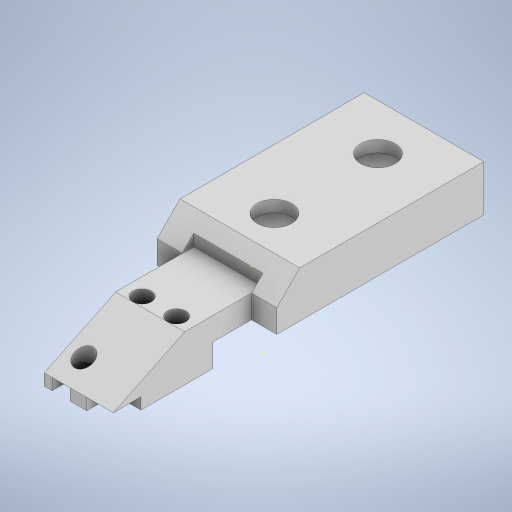
# Autodesk Inventor part: electrodeholder_screwon_4
Saved by Autodesk Inventor 2023 (Build 270158000, 158)
## iProperties
Created: 2022-09-20
Part Number: electrodeholder_screwon_4
Material: Generic
Document SubType Name: Modeling
Designer: Connor
Density: 1 g/cm^3
Appearance: Default
Author: Connor
Autodesk Inventor part; units mm, degrees
ref_plane "YZ Plane" through (0, 0, 0) normal (1, 0, 0) x (0, 1, 0)
ref_plane "XZ Plane" through (0, 0, 0) normal (0, 1, 0) x (-1, 0, 0)
ref_plane "XY Plane" through (0, 0, 0) normal (0, 0, 1) x (1, 0, 0)
sketch "Sketch1" plane through (0, 0, 0) normal (0, 1, 0) x (-1, 0, 0)
  line L0 (0, 0) -> (12.7, 0)
  line L1 (12.7, 0) -> (12.7, -25.4)
  line L2 (12.7, -25.4) -> (0, -25.4)
  line L3 (0, -25.4) -> (0, 0)
  dimension "d0" = 12.7
  dimension "d1" = 25.4
  constraints: 8 end point, 2 parallel, 1 horizontal, 1 perpendicular
  measures "d0" distance of L1.end L2.end
  measures "d1" distance of L0.end L1.end
sketch "Sketch1 outline for Extrusion1" plane through (0, 0, 0) normal (0, 1, 0) x (-1, 0, 0)
  line L0 (0, 0) -> (0, -25.4)
  line L1 (12.7, 0) -> (0, 0)
  line L2 (12.7, -25.4) -> (12.7, 0)
  line L3 (0, -25.4) -> (12.7, -25.4)
extrude "Extrusion1" add sketch "Sketch1 outline for Extrusion1" along normal blind 7.62
sketch "Sketch2" plane through (0, 0, 0) normal (1, 0, 0) x (0, 0, -1)
  line L0 (25.4, 7.62) -> (0, 7.62) projected
  line L1 (25.4, 0) -> (0, 0) projected
  line L2 (0, 7.62) -> (7.62, 7.62)
  line L3 (7.62, 7.62) -> (7.62, 0)
  line L4 (7.62, 0) -> (0, 0)
  line L5 (0, 0) -> (0, 7.62)
  line L6 (0, 0) -> (7.62, 7.62)
  dimension "d4" = 7.62
  constraints: 10 end point, 2 parallel, 1 horizontal, 1 perpendicular, 1 point on line
  measures "d4" distance of L3.end L4.end
sketch "Sketch2 outline for Extrusion2" plane through (0, 0, 0) normal (1, 0, 0) x (0, 0, -1)
  line L0 (0, 7.62) -> (0, 0)
  line L1 (7.62, 7.62) -> (0, 7.62)
  line L2 (0, 0) -> (7.62, 7.62)
extrude "Extrusion2" cut sketch "Sketch2 outline for Extrusion2" against normal blind 25.4
sketch "Sketch3" plane through (0, 0, 0) normal (0, -1, 0) x (1, 0, 0)
  line L0 (-12.7, -25.4) -> (-12.7, 0) projected
  line L1 (0, 0) -> (-12.7, 0)
  line L2 (-12.7, 0) -> (-12.7, -8.89)
  line L3 (-12.7, -8.89) -> (0, -8.89)
  line L4 (0, -8.89) -> (0, 0)
  circle A0 centre (-6.35, -8.89) radius 4.445
  dimension "d7" = 8.89
  dimension "d8" = 8.89
  constraints: 8 end point, 2 parallel, 1 centre point, 1 horizontal, 1 midpoint, 1 perpendicular, 1 point on line
  measures "d7" distance of L2.end L1.end
  measures "d8" diameter of A0
sketch "Sketch3 outline for Extrusion3" plane through (0, 0, 0) normal (0, -1, 0) x (1, 0, 0)
  circle A0 centre (-6.35, -8.89) radius 4.445
extrude "Extrusion3" cut sketch "Sketch3 outline for Extrusion3" against normal blind 3.81
sketch "Sketch4" plane through (0, 0, 0) normal (0, -1, 0) x (1, 0, 0)
  circle A0 centre (-6.35, -8.89) radius 4.445 projected
  line L0 (-6.35, -8.89) -> (-6.35, -20.32)
  circle A1 centre (-6.35, -20.32) radius 4.445
  point P0 (0, 0)
  dimension "d11" = 11.43
  dimension "d12" = 8.89
  constraints: 2 end point, 1 centre point, 1 coincident, 1 vertical
  measures "d11" distance of L0.start L0.end
  measures "d12" diameter of A1
sketch "Sketch4 outline for Extrusion4" plane through (0, 0, 0) normal (0, -1, 0) x (1, 0, 0)
  circle A0 centre (-6.35, -20.32) radius 4.445
extrude "Extrusion4" cut sketch "Sketch4 outline for Extrusion4" against normal blind 2.54
sketch "Sketch6" plane through (0, 0, -25.4) normal (1, 0, 0) x (0, 0, -1)
  line L0 (-25.4, 0) -> (-22.86, 0)
  line L1 (-22.86, 0) -> (-22.86, 2.54)
  line L2 (-22.86, 2.54) -> (-25.4, 2.54)
  line L3 (-25.4, 2.54) -> (-25.4, 0)
  dimension "d18" = 2.54
  dimension "d19" = 2.54
  constraints: 8 end point, 2 parallel, 1 horizontal, 1 perpendicular
  measures "d18" distance of L2.end L1.end
  measures "d19" distance of L1.end L0.end
sketch "Sketch6 outline for Extrusion6" plane through (0, 0, -25.4) normal (1, 0, 0) x (0, 0, -1)
  line L0 (-25.4, 0) -> (-22.86, 0)
  line L1 (-25.4, 2.54) -> (-25.4, 0)
  line L2 (-22.86, 2.54) -> (-25.4, 2.54)
  line L3 (-22.86, 0) -> (-22.86, 2.54)
extrude "Extrusion6" cut sketch "Sketch6 outline for Extrusion6" against normal blind 25.4
sketch "Sketch7" plane through (0, 0, -2.54) normal (0, 0, 1) x (1, 0, 0)
  line L0 (-12.7, 0) -> (-12.7, 2.54) projected
  line L1 (0, 0) -> (-12.7, 0) projected
  line L2 (0, 2.54) -> (0, 0) projected
  line L3 (-12.7, 2.54) -> (0, 2.54) projected
sketch "Sketch7 outline for Extrusion7" plane through (0, 0, -2.54) normal (0, 0, 1) x (1, 0, 0)
  line L0 (-12.7, 0) -> (0, 0)
  line L1 (-12.7, 2.54) -> (-12.7, 0)
  line L2 (0, 2.54) -> (-12.7, 2.54)
  line L3 (0, 0) -> (0, 2.54)
extrude "Extrusion7" add sketch "Sketch7 outline for Extrusion7" along normal blind 12.7
sketch "Sketch13" plane through (0, 0, 0) normal (0, -1, 0) x (1, 0, 0)
  line L0 (-12.7, -2.54) -> (-12.7, -7.62) projected
  line L1 (0, -2.54) -> (0, 10.16) projected
  line L2 (-12.7, -2.54) -> (0, -2.54)
  line L3 (0, -2.54) -> (0, 10.16)
  line L4 (0, 10.16) -> (-12.7, 10.16)
  line L5 (-12.7, 10.16) -> (-12.7, -2.54)
  line L6 (0, -7.62) -> (0, -2.54) projected
  line L7 (-12.7, 10.16) -> (0, 10.16) projected
  line L8 (0, -2.54) -> (-2.54, -2.54)
  line L9 (-2.54, -2.54) -> (-2.54, 10.16)
  line L10 (-2.54, 10.16) -> (0, 10.16)
  line L11 (0, 10.16) -> (0, -2.54)
  line L12 (-12.7, -2.54) -> (-10.16, -2.54)
  line L13 (-10.16, -2.54) -> (-10.16, 10.16)
  line L14 (-10.16, 10.16) -> (-12.7, 10.16)
  line L15 (-12.7, 10.16) -> (-12.7, -2.54)
  point P0 (0, 0)
  dimension "d43" = 2.54
  dimension "d44" = 2.54
  constraints: 24 end point, 6 parallel, 3 horizontal, 3 perpendicular, 2 point on line
  measures "d43" distance of L9.end L10.end
  measures "d44" distance of L14.end L13.end
sketch "Sketch13 outline for Extrusion13" plane through (0, 0, 0) normal (0, -1, 0) x (1, 0, 0)
  line L0 (-10.16, -2.54) -> (-10.16, 10.16)
  line L1 (-12.7, -2.54) -> (-10.16, -2.54)
  line L2 (-12.7, 10.16) -> (-12.7, -2.54)
  line L3 (-10.16, 10.16) -> (-12.7, 10.16)
  line L4 (-2.54, 10.16) -> (-2.54, -2.54)
  line L5 (0, 10.16) -> (-2.54, 10.16)
  line L6 (0, -2.54) -> (0, 10.16)
  line L7 (-2.54, -2.54) -> (0, -2.54)
extrude "Extrusion13" cut sketch "Sketch13 outline for Extrusion13" against normal blind 2.54
sketch "Sketch18" plane through (0, 0, 0) normal (0, -1, 0) x (1, 0, 0)
  line L0 (-2.54, 10.16) -> (-10.16, 10.16) projected
  line L1 (-10.16, -2.54) -> (-10.16, 10.16) projected
  line L2 (-2.54, 10.16) -> (-10.16, 10.16)
  line L3 (-10.16, 10.16) -> (-10.16, 2.54)
  line L4 (-10.16, 2.54) -> (-2.54, 2.54)
  line L5 (-2.54, 2.54) -> (-2.54, 10.16)
  line L6 (-10.16, -2.54) -> (-2.54, -2.54) projected
  line L7 (-6.35, -2.54) -> (-6.35, 10.16)
  line L8 (-6.35, -2.54) -> (-2.54, -2.54)
  line L9 (-2.54, -2.54) -> (-4.445, -2.54)
  line L10 (-4.445, 10.16) -> (-4.445, -2.54)
  line L11 (-10.16, -2.54) -> (-6.35, -2.54)
  line L12 (-8.255, -2.54) -> (-8.255, 10.16)
  circle A0 centre (-4.445, 3.81) radius 1.016
  circle A1 centre (-8.255, 3.81) radius 1.016
  point P0 (0, 0)
  dimension "d63" = 7.62
  dimension "d64" = 2.032
  dimension "d65" = 2.032
  constraints: 20 end point, 6 midpoint, 4 perpendicular, 3 point on line, 2 centre point, 2 horizontal, 2 parallel
  measures "d63" distance of L3.end L2.end
  measures "d64" diameter of A0
  measures "d65" diameter of A1
sketch "Sketch18 outline for Extrusion18" plane through (0, 0, 0) normal (0, -1, 0) x (1, 0, 0)
  circle A0 centre (-8.255, 3.81) radius 1.016
  circle A1 centre (-4.445, 3.81) radius 1.016
extrude "Extrusion18" cut sketch "Sketch18 outline for Extrusion18" against normal blind 25.4
sketch "Sketch19" plane through (0, 0, 0) normal (0, -1, 0) x (1, 0, 0)
  circle A0 centre (-4.445, 3.81) radius 1.016
  line L0 (-2.54, 10.16) -> (-10.16, 10.16)
  line L1 (-5.461, 3.81) -> (-7.285663, 3.81)
  line L2 (-7.285663, 3.81) -> (-7.285663, 10.16)
  line L3 (-7.285663, 10.16) -> (-5.461, 10.16)
  line L4 (-5.461, 10.16) -> (-5.461, 3.81)
  point P0 (0, 0)
  constraints: 8 end point, 2 parallel, 1 horizontal, 1 horizontal alignment, 1 perpendicular, 1 point on line, 1 other
sketch "Sketch19 outline for Extrusion19" plane through (0, 0, 0) normal (0, -1, 0) x (1, 0, 0)
  line L0 (-5.461, 3.81) -> (-5.461, 10.16)
  line L1 (-7.285663, 3.81) -> (-5.461, 3.81)
  line L2 (-7.285663, 10.16) -> (-7.285663, 3.81)
  line L3 (-5.461, 10.16) -> (-7.285663, 10.16)
extrude "Extrusion19" add sketch "Sketch19 outline for Extrusion19" along normal blind 2.54
sketch "Sketch20" plane through (0, 0, 0) normal (0, -1, 0) x (1, 0, 0)
  line L0 (-5.461, 3.81) -> (-7.239, 3.81) projected
  line L1 (-5.461, 3.81) -> (-7.239, 3.81)
  line L2 (-7.239, 3.81) -> (-7.239, 2.54)
  line L3 (-7.239, 2.54) -> (-5.461, 2.54)
  line L4 (-5.461, 2.54) -> (-5.461, 3.81)
  point P0 (0, 0)
  dimension "d70" = 1.27
  constraints: 8 end point, 2 parallel, 1 horizontal, 1 perpendicular
  measures "d70" distance of L2.end L1.end
sketch "Sketch20 outline for Extrusion20" plane through (0, 0, 0) normal (0, -1, 0) x (1, 0, 0)
  line L0 (-5.461, 2.54) -> (-5.461, 3.81)
  line L1 (-7.239, 2.54) -> (-5.461, 2.54)
  line L2 (-7.239, 3.81) -> (-7.239, 2.54)
  line L3 (-5.461, 3.81) -> (-7.239, 3.81)
extrude "Extrusion20" add sketch "Sketch20 outline for Extrusion20" along normal blind 2.54
sketch "Sketch21" plane through (-10.16, 2.54, 10.16) normal (0, 1, 0) x (1, 0, 0)
  circle A0 centre (1.905, 6.35) radius 1.016 projected
  circle A1 centre (5.715, 6.35) radius 1.016 projected
  line L0 (0, 12.7) -> (0, 0) projected
  line L1 (7.62, 0) -> (0, 0) projected
  line L2 (7.62, 0) -> (7.62, 12.7) projected
  line L3 (0, 12.7) -> (7.62, 12.7) projected
  point P0 (10.16, 10.16)
sketch "Sketch21 outline for Extrusion21" plane through (-10.16, 2.54, 10.16) normal (0, 1, 0) x (1, 0, 0)
  line L0 (7.62, 0) -> (7.62, 12.7)
  line L1 (0, 0) -> (7.62, 0)
  line L2 (7.62, 12.7) -> (0, 12.7)
  line L3 (0, 12.7) -> (0, 0)
  circle A0 centre (1.905, 6.35) radius 1.016
  circle A1 centre (5.715, 6.35) radius 1.016
extrude "Extrusion21" add sketch "Sketch21 outline for Extrusion21" along normal blind 1.27
sketch "Sketch22" plane through (-2.54, 2.54, -2.54) normal (0, 0, -1) x (-1, 0, 0)
  line L0 (7.62, 0) -> (0, 0) projected
  line L1 (7.62, 0) -> (7.62, 1.27) projected
  line L2 (0, 1.27) -> (7.62, 1.27) projected
  line L3 (0, 0) -> (0, 1.27) projected
  point P0 (-2.54, -2.54)
sketch "Sketch22 outline for Extrusion22" plane through (-2.54, 2.54, -2.54) normal (0, 0, -1) x (-1, 0, 0)
  line L0 (7.62, 0) -> (7.62, 1.27)
  line L1 (0, 0) -> (7.62, 0)
  line L2 (0, 1.27) -> (0, 0)
  line L3 (7.62, 1.27) -> (0, 1.27)
extrude "Extrusion22" add sketch "Sketch22 outline for Extrusion22" along normal blind 5.08
sketch "Sketch23" plane through (-6.35, 2.54, -8.89) normal (0, -1, 0) x (1, 0, 0)
  circle A0 centre (0, 0) radius 4.445
  point P0 (6.35, 8.89)
  constraints: 1 centre point
sketch "Sketch23 outline for Extrusion23" plane through (-6.35, 2.54, -8.89) normal (0, -1, 0) x (1, 0, 0)
  circle A0 centre (0, 0) radius 4.445
extrude "Extrusion23" cut sketch "Sketch23 outline for Extrusion23" against normal blind 1.27
sketch "Sketch24" plane through (-10.16, 3.81, 10.16) normal (0, 1, 0) x (1, 0, 0)
  line L0 (0, 0) -> (0, 13.97) projected
  line L1 (0, 0) -> (7.62, 0) projected
  line L2 (7.62, 0) -> (7.62, 13.97) projected
  line L3 (0, 13.97) -> (7.62, 13.97) projected
  circle A0 centre (5.715, 6.35) radius 1.016 projected
  circle A1 centre (1.905, 6.35) radius 1.016 projected
  point P0 (10.16, 10.16)
sketch "Sketch24 outline for Extrusion24" plane through (-10.16, 3.81, 10.16) normal (0, 1, 0) x (1, 0, 0)
  line L0 (7.62, 0) -> (7.62, 13.97)
  line L1 (0, 0) -> (7.62, 0)
  line L2 (7.62, 13.97) -> (0, 13.97)
  line L3 (0, 13.97) -> (0, 0)
  circle A0 centre (1.905, 6.35) radius 1.016
  circle A1 centre (5.715, 6.35) radius 1.016
extrude "Extrusion24" cut sketch "Sketch24 outline for Extrusion24" against normal blind 2.54
sketch "Sketch26" plane through (0, 0, 10.16) normal (0, 0, 1) x (1, 0, 0)
  line L0 (-2.54, 1.27) -> (-10.16, 1.27)
  line L1 (-10.16, 0) -> (-10.16, 1.27)
  line L2 (-10.16, 0) -> (-7.285663, 0)
  line L3 (-7.285663, 0) -> (-7.285663, -2.54)
  line L4 (-5.461, -2.54) -> (-7.285663, -2.54)
  line L5 (-5.461, 0) -> (-5.461, -2.54)
  line L6 (-5.461, 0) -> (-2.54, 0)
  line L7 (-2.54, 0) -> (-2.54, 1.27)
  point P0 (0, 0)
sketch "Sketch26 outline for Extrusion26" plane through (0, 0, 10.16) normal (0, 0, 1) x (1, 0, 0)
  line L0 (-5.461, 0) -> (-2.54, 0)
  line L1 (-5.461, -2.54) -> (-5.461, 0)
  line L2 (-7.285663, -2.54) -> (-5.461, -2.54)
  line L3 (-7.285663, 0) -> (-7.285663, -2.54)
  line L4 (-10.16, 0) -> (-7.285663, 0)
  line L5 (-10.16, 1.27) -> (-10.16, 0)
  line L6 (-2.54, 1.27) -> (-10.16, 1.27)
  line L7 (-2.54, 0) -> (-2.54, 1.27)
extrude "Extrusion26" add sketch "Sketch26 outline for Extrusion26" along normal blind 2.54
sketch "Sketch27" plane through (0, 0, -25.4) normal (1, 0, 0) x (0, 0, -1)
  line L0 (-22.86, 2.54) -> (-22.86, 0) projected
  line L1 (-22.86, 0) -> (0, 0) projected
  line L2 (0, 0) -> (0, 7.62) projected
  line L3 (-17.78, 7.62) -> (0, 7.62) projected
  line L4 (-17.78, 7.62) -> (-22.86, 2.54) projected
  point P0 (-25.4, 0)
sketch "Sketch27 outline for Extrusion27" plane through (0, 0, -25.4) normal (1, 0, 0) x (0, 0, -1)
  line L0 (-17.78, 7.62) -> (-22.86, 2.54)
  line L1 (0, 7.62) -> (-17.78, 7.62)
  line L2 (0, 0) -> (0, 7.62)
  line L3 (-22.86, 0) -> (0, 0)
  line L4 (-22.86, 2.54) -> (-22.86, 0)
extrude "Extrusion27" add sketch "Sketch27 outline for Extrusion27" along normal blind 1.27
sketch "Sketch28" plane through (-12.7, 0, -25.4) normal (-1, 0, 0) x (0, 0, 1)
  line L0 (0, 7.62) -> (17.78, 7.62) projected
  line L1 (0, 0) -> (0, 7.62) projected
  line L2 (0, 0) -> (22.86, 0) projected
  line L3 (22.86, 0) -> (22.86, 2.54) projected
  line L4 (22.86, 2.54) -> (17.78, 7.62) projected
  point P0 (25.4, 0)
sketch "Sketch28 outline for Extrusion28" plane through (-12.7, 0, -25.4) normal (-1, 0, 0) x (0, 0, 1)
  line L0 (0, 0) -> (22.86, 0)
  line L1 (0, 7.62) -> (0, 0)
  line L2 (17.78, 7.62) -> (0, 7.62)
  line L3 (22.86, 2.54) -> (17.78, 7.62)
  line L4 (22.86, 0) -> (22.86, 2.54)
extrude "Extrusion28" add sketch "Sketch28 outline for Extrusion28" along normal blind 1.27
sketch "Sketch29" plane through (0, -2.54, 0) normal (0, -1, 0) x (1, 0, 0)
  line L0 (-7.285663, 3.81) -> (-7.285663, 12.7)
  line L1 (-7.285663, 3.81) -> (-7.239, 3.81)
  line L2 (-7.239, 3.81) -> (-7.239, 2.54)
  line L3 (-7.239, 2.54) -> (-5.461, 2.54)
  line L4 (-5.461, 2.54) -> (-5.461, 12.7)
  line L5 (-7.285663, 12.7) -> (-5.461, 12.7)
  point P0 (0, 0)
sketch "Sketch29 outline for Extrusion29" plane through (0, -2.54, 0) normal (0, -1, 0) x (1, 0, 0)
  line L0 (-7.239, 3.81) -> (-7.239, 2.54)
  line L1 (-7.285663, 3.81) -> (-7.239, 3.81)
  line L2 (-7.285663, 12.7) -> (-7.285663, 3.81)
  line L3 (-5.461, 12.7) -> (-7.285663, 12.7)
  line L4 (-5.461, 2.54) -> (-5.461, 12.7)
  line L5 (-7.239, 2.54) -> (-5.461, 2.54)
extrude "Extrusion29" cut sketch "Sketch29 outline for Extrusion29" against normal blind 1.27
sketch "Sketch31" plane through (0, 7.62, 0) normal (0, 1, 0) x (1, 0, 0)
  point P0 (0, 0)
sketch "Sketch32" plane through (0, 7.62, 0) normal (0, 1, 0) x (1, 0, 0)
  point P0 (0, 0)
sketch "Sketch33" plane through (0, 7.62, 0) normal (0, 1, 0) x (1, 0, 0)
  line L0 (-13.97, 7.62) -> (1.27, 7.62) projected
  line L1 (1.27, 25.4) -> (1.27, 7.62) projected
  line L2 (-13.97, 25.4) -> (1.27, 25.4) projected
  line L3 (-13.97, 7.62) -> (-13.97, 25.4) projected
  point P0 (0, 0)
sketch "Sketch33 outline for Extrusion30" plane through (0, 7.62, 0) normal (0, 1, 0) x (1, 0, 0)
  line L0 (-13.97, 25.4) -> (-13.97, 7.62)
  line L1 (1.27, 25.4) -> (-13.97, 25.4)
  line L2 (1.27, 7.62) -> (1.27, 25.4)
  line L3 (-13.97, 7.62) -> (1.27, 7.62)
extrude "Extrusion30" add sketch "Sketch33 outline for Extrusion30" along normal blind 5.08
sketch "Sketch35" plane through (1.27, 0, -25.4) normal (1, 0, 0) x (0, 0, -1)
  point P0 (-25.4, 0)
sketch "Sketch36" plane through (1.27, 0, -25.4) normal (1, 0, 0) x (0, 0, -1)
  line L0 (-22.86, 2.54) -> (-22.86, 0) projected
  line L1 (-22.86, 0) -> (0, 0) projected
  line L2 (0, 0) -> (0, 12.7) projected
  line L3 (-17.78, 12.7) -> (0, 12.7) projected
  line L4 (-17.78, 7.62) -> (-17.78, 12.7) projected
  line L5 (-17.78, 7.62) -> (-22.86, 2.54) projected
  point P0 (-25.4, 0)
sketch "Sketch36 outline for Extrusion33" plane through (1.27, 0, -25.4) normal (1, 0, 0) x (0, 0, -1)
  line L0 (-17.78, 7.62) -> (-22.86, 2.54)
  line L1 (-17.78, 12.7) -> (-17.78, 7.62)
  line L2 (0, 12.7) -> (-17.78, 12.7)
  line L3 (0, 0) -> (0, 12.7)
  line L4 (-22.86, 0) -> (0, 0)
  line L5 (-22.86, 2.54) -> (-22.86, 0)
extrude "Extrusion33" cut sketch "Sketch36 outline for Extrusion33" against normal blind 0.254
sketch "Sketch37" plane through (-13.97, 0, -25.4) normal (-1, 0, 0) x (0, 0, 1)
  line L0 (22.86, 0) -> (22.86, 2.54) projected
  line L1 (22.86, 2.54) -> (17.78, 7.62) projected
  line L2 (17.78, 7.62) -> (17.78, 12.7) projected
  line L3 (0, 12.7) -> (17.78, 12.7) projected
  line L4 (0, 0) -> (0, 12.7) projected
  line L5 (0, 0) -> (22.86, 0) projected
  point P0 (25.4, 0)
sketch "Sketch37 outline for Extrusion34" plane through (-13.97, 0, -25.4) normal (-1, 0, 0) x (0, 0, 1)
  line L0 (0, 0) -> (22.86, 0)
  line L1 (0, 12.7) -> (0, 0)
  line L2 (17.78, 12.7) -> (0, 12.7)
  line L3 (17.78, 7.62) -> (17.78, 12.7)
  line L4 (22.86, 2.54) -> (17.78, 7.62)
  line L5 (22.86, 0) -> (22.86, 2.54)
extrude "Extrusion34" cut sketch "Sketch37 outline for Extrusion34" against normal blind 0.254
sketch "Sketch38" plane through (0, 0, 0) normal (0, -1, 0) x (1, 0, 0)
  line L0 (-10.16, -2.54) -> (-10.16, 12.7)
  line L1 (-2.54, -2.54) -> (-2.54, 12.7)
  line L2 (-10.16, 12.7) -> (-2.54, 12.7)
  line L3 (-2.54, 12.7) -> (-2.54, 1.734585)
  line L4 (-2.54, 1.734585) -> (-10.16, 1.734585)
  line L5 (-10.16, 1.734585) -> (-10.16, 12.7)
  circle A0 centre (-6.35, -8.89) radius 4.445
  circle A1 centre (-6.35, -20.32) radius 4.445
  line L6 (-13.716, -2.54) -> (-13.716, -25.4)
  line L7 (1.016, -25.4) -> (-13.716, -25.4)
  line L8 (1.016, -25.4) -> (1.016, -2.54)
  line L9 (1.016, -2.54) -> (-2.54, -2.54)
  line L10 (-2.54, -2.54) -> (-2.54, 12.7)
  line L11 (-5.461, 12.7) -> (-2.54, 12.7)
  line L12 (-5.461, 12.7) -> (-5.461, 3.81)
  circle A2 centre (-4.445, 3.81) radius 1.016
  line L13 (-5.461, 3.81) -> (-5.461, 2.54)
  line L14 (-5.461, 2.54) -> (-7.239, 2.54)
  line L15 (-7.239, 2.54) -> (-7.239, 3.81)
  arc A3 (-7.285663, 4.114372) -> (-7.239, 3.81) centre (-8.255, 3.81) ccw
  line L16 (-7.285663, 4.114372) -> (-7.285663, 12.7)
  line L17 (-10.16, 12.7) -> (-7.285663, 12.7)
  line L18 (-10.16, 12.7) -> (-10.16, -2.54)
  line L19 (-10.16, -2.54) -> (-13.716, -2.54)
  point P0 (0, 0)
  constraints: 8 end point, 2 parallel, 1 horizontal, 1 horizontal alignment, 1 perpendicular, 1 point on line
sketch "Sketch38 outline for Extrusion35" plane through (0, 0, 0) normal (0, -1, 0) x (1, 0, 0)
  line L0 (-5.461, 2.54) -> (-7.239, 2.54)
  line L1 (-5.461, 3.81) -> (-5.461, 2.54)
  line L2 (-5.461, 12.7) -> (-5.461, 3.81)
  line L3 (-2.54, 12.7) -> (-5.461, 12.7)
  line L4 (-2.54, 1.734585) -> (-2.54, 12.7)
  line L5 (-10.16, 1.734585) -> (-2.54, 1.734585)
  line L6 (-10.16, 12.7) -> (-10.16, 1.734585)
  line L7 (-7.285663, 12.7) -> (-10.16, 12.7)
  line L8 (-7.285663, 4.114372) -> (-7.285663, 12.7)
  arc A0 (-7.239, 3.81) -> (-7.285663, 4.114372) centre (-8.255, 3.81) cw
  line L9 (-7.239, 2.54) -> (-7.239, 3.81)
  arc A1 (-5.461, 3.81) -> (-3.429, 3.81) centre (-4.445, 3.81) ccw
  arc A2 (-3.429, 3.81) -> (-5.461, 3.81) centre (-4.445, 3.81) ccw
extrude "Extrusion35" add sketch "Sketch38 outline for Extrusion35" along normal blind 1.27
sketch "Sketch39" plane through (0, -1.27, 0) normal (0, -1, 0) x (1, 0, 0)
  line L0 (-2.54, 12.7) -> (-10.16, 12.7)
  line L1 (-5.462315, 3.81) -> (-7.300103, 3.81)
  line L2 (-7.300103, 3.81) -> (-7.300103, 12.7)
  line L3 (-7.300103, 12.7) -> (-5.462315, 12.7)
  line L4 (-5.462315, 12.7) -> (-5.462315, 3.81)
  point P0 (0, 0)
  constraints: 8 end point, 2 parallel, 1 horizontal, 1 perpendicular, 1 point on line
sketch "Sketch39 outline for Extrusion36" plane through (0, -1.27, 0) normal (0, -1, 0) x (1, 0, 0)
  line L0 (-7.300103, 3.81) -> (-5.462315, 3.81)
  line L1 (-7.300103, 12.7) -> (-7.300103, 3.81)
  line L2 (-5.462315, 12.7) -> (-7.300103, 12.7)
  line L3 (-5.462315, 3.81) -> (-5.462315, 12.7)
extrude "Extrusion36" add sketch "Sketch39 outline for Extrusion36" along normal blind 1.27
sketch "Sketch40" plane through (0, -1.27, 0) normal (0, -1, 0) x (1, 0, 0)
  circle A0 centre (-4.445, 3.81) radius 1.016
  line L0 (-5.461, 3.81) -> (-7.300103, 3.81)
  line L1 (-7.300103, 3.81) -> (-7.300103, 2.501434)
  line L2 (-7.300103, 2.501434) -> (-5.461, 2.501434)
  line L3 (-5.461, 2.501434) -> (-5.461, 3.81)
  point P0 (0, 0)
  constraints: 8 end point, 2 parallel, 1 horizontal, 1 horizontal alignment, 1 perpendicular, 1 other
sketch "Sketch40 outline for Extrusion37" plane through (0, -1.27, 0) normal (0, -1, 0) x (1, 0, 0)
  line L0 (-7.300103, 2.501434) -> (-5.461, 2.501434)
  line L1 (-7.300103, 3.81) -> (-7.300103, 2.501434)
  line L2 (-5.461, 3.81) -> (-7.300103, 3.81)
  line L3 (-5.461, 2.501434) -> (-5.461, 3.81)
extrude "Extrusion37" add sketch "Sketch40 outline for Extrusion37" along normal blind 1.27
sketch "Sketch41" plane through (-10.16, 1.27, 10.16) normal (0, 1, 0) x (1, 0, 0)
  line L0 (0, -2.54) -> (0, 8.425415)
  line L1 (7.62, 13.97) -> (7.62, 12.7)
  line L2 (0, 8.425415) -> (7.62, 8.425415)
  line L3 (7.62, 8.425415) -> (7.62, 13.97)
  line L4 (7.62, 13.97) -> (0, 13.97)
  line L5 (0, 13.97) -> (0, 8.425415)
  point P0 (10.16, 10.16)
  constraints: 8 end point, 2 parallel, 1 horizontal, 1 perpendicular
sketch "Sketch41 outline for Extrusion38" plane through (-10.16, 1.27, 10.16) normal (0, 1, 0) x (1, 0, 0)
  line L0 (0, 8.425415) -> (7.62, 8.425415)
  line L1 (0, 13.97) -> (0, 8.425415)
  line L2 (7.62, 13.97) -> (0, 13.97)
  line L3 (7.62, 12.7) -> (7.62, 13.97)
  line L4 (7.62, 8.425415) -> (7.62, 12.7)
extrude "Extrusion38" add sketch "Sketch41 outline for Extrusion38" along normal blind 1.27
sketch "Sketch42" plane through (-10.16, 1.27, 10.16) normal (0, 1, 0) x (1, 0, 0)
  line L0 (0, 8.425415) -> (7.62, 8.425415)
  line L1 (7.62, 8.425415) -> (7.62, -2.54)
  line L2 (0, 8.425415) -> (7.62, 8.425415)
  line L3 (7.62, 8.425415) -> (7.62, 7.530789)
  line L4 (7.62, 7.530789) -> (0, 7.530789)
  line L5 (0, 7.530789) -> (0, 8.425415)
  point P0 (10.16, 10.16)
  constraints: 8 end point, 2 parallel, 1 horizontal, 1 perpendicular, 1 point on line
sketch "Sketch42 outline for Extrusion39" plane through (-10.16, 1.27, 10.16) normal (0, 1, 0) x (1, 0, 0)
  line L0 (0, 8.425415) -> (0, 7.530789)
  line L1 (7.62, 8.425415) -> (0, 8.425415)
  line L2 (7.62, 7.530789) -> (7.62, 8.425415)
  line L3 (0, 7.530789) -> (7.62, 7.530789)
extrude "Extrusion39" add sketch "Sketch42 outline for Extrusion39" along normal blind 1.27
sketch "Sketch43" plane through (-10.16, 1.27, 10.16) normal (0, 1, 0) x (1, 0, 0)
  circle A0 centre (1.905, 6.35) radius 1.016
  circle A1 centre (5.715, 6.35) radius 1.016
  line L0 (7.62, 7.530789) -> (0, 7.530789)
  line L1 (0, 7.530789) -> (0, -2.54)
  line L2 (7.62, -2.54) -> (0, -2.54)
  line L3 (7.62, 7.530789) -> (7.62, -2.54)
  point P0 (10.16, 10.16)
sketch "Sketch43 outline for Extrusion40" plane through (-10.16, 1.27, 10.16) normal (0, 1, 0) x (1, 0, 0)
  line L0 (7.62, -2.54) -> (7.62, 7.530789)
  line L1 (0, -2.54) -> (7.62, -2.54)
  line L2 (7.62, 7.530789) -> (0, 7.530789)
  line L3 (0, 7.530789) -> (0, -2.54)
  circle A0 centre (1.905, 6.35) radius 1.016
  circle A1 centre (5.715, 6.35) radius 1.016
extrude "Extrusion40" add sketch "Sketch43 outline for Extrusion40" along normal blind 1.27
sketch "Sketch44" plane through (1.016, 0, -25.4) normal (1, 0, 0) x (0, 0, -1)
  line L0 (0, 12.7) -> (-17.78, 12.7) projected
  line L1 (-17.78, 12.7) -> (-17.78, 7.62) projected
  line L2 (0, 12.7) -> (-17.78, 12.7)
  line L3 (-17.78, 12.7) -> (-17.78, 10.16)
  line L4 (-17.78, 10.16) -> (0, 10.16)
  line L5 (0, 10.16) -> (0, 12.7)
  point P0 (-25.4, 0)
  constraints: 8 end point, 2 parallel, 1 horizontal, 1 midpoint, 1 perpendicular
sketch "Sketch44 outline for Extrusion41" plane through (1.016, 0, -25.4) normal (1, 0, 0) x (0, 0, -1)
  line L0 (0, 10.16) -> (0, 12.7)
  line L1 (-17.78, 10.16) -> (0, 10.16)
  line L2 (-17.78, 12.7) -> (-17.78, 10.16)
  line L3 (0, 12.7) -> (-17.78, 12.7)
extrude "Extrusion41" cut sketch "Sketch44 outline for Extrusion41" against normal blind 2540
sketch "Sketch45" plane through (1.016, 0, -25.4) normal (1, 0, 0) x (0, 0, -1)
  line L0 (0, 10.16) -> (-17.78, 10.16) projected
  line L1 (-17.78, 7.62) -> (-17.78, 10.16) projected
  line L2 (-22.86, 2.54) -> (-17.78, 7.62) projected
  line L3 (-22.86, 0) -> (-22.86, 2.54) projected
  line L4 (0, 0) -> (-22.86, 0) projected
  line L5 (0, 10.16) -> (0, 0) projected
  point P0 (-25.4, 0)
sketch "Sketch45 outline for Extrusion42" plane through (1.016, 0, -25.4) normal (1, 0, 0) x (0, 0, -1)
  line L0 (0, 0) -> (0, 10.16)
  line L1 (-22.86, 0) -> (0, 0)
  line L2 (-22.86, 2.54) -> (-22.86, 0)
  line L3 (-17.78, 7.62) -> (-22.86, 2.54)
  line L4 (-17.78, 10.16) -> (-17.78, 7.62)
  line L5 (0, 10.16) -> (-17.78, 10.16)
extrude "Extrusion42" cut sketch "Sketch45 outline for Extrusion42" against normal blind 0.762
sketch "Sketch46" plane through (-13.716, 0, -25.4) normal (-1, 0, 0) x (0, 0, 1)
  line L0 (17.78, 10.16) -> (0, 10.16) projected
  line L1 (0, 0) -> (0, 10.16) projected
  line L2 (22.86, 0) -> (0, 0) projected
  line L3 (22.86, 2.54) -> (22.86, 0) projected
  line L4 (17.78, 7.62) -> (22.86, 2.54) projected
  line L5 (17.78, 10.16) -> (17.78, 7.62) projected
  point P0 (25.4, 0)
sketch "Sketch46 outline for Extrusion43" plane through (-13.716, 0, -25.4) normal (-1, 0, 0) x (0, 0, 1)
  line L0 (17.78, 7.62) -> (17.78, 10.16)
  line L1 (22.86, 2.54) -> (17.78, 7.62)
  line L2 (22.86, 0) -> (22.86, 2.54)
  line L3 (0, 0) -> (22.86, 0)
  line L4 (0, 10.16) -> (0, 0)
  line L5 (17.78, 10.16) -> (0, 10.16)
extrude "Extrusion43" cut sketch "Sketch46 outline for Extrusion43" against normal blind 0.762
sketch "Sketch47" plane through (-2.54, 0, 1.734585) normal (1, 0, 0) x (0, 0, -1)
  line L0 (-2.422442, -1.27) -> (-10.965415, -1.27)
  line L1 (-10.965415, -1.27) -> (-3.091415, 2.54)
  line L2 (-3.091415, -1.27) -> (-3.091415, 2.54)
  line L3 (-10.965415, 2.54) -> (4.274585, 2.54)
  line L4 (-10.965415, 2.54) -> (-3.091415, 2.54)
  line L5 (-3.091415, 2.54) -> (-3.091415, -2.54)
  line L6 (-3.091415, -2.54) -> (-10.965415, -2.54)
  line L7 (-10.965415, -2.54) -> (-10.965415, 2.54)
  point P0 (1.734585, 0)
  constraints: 10 end point, 2 parallel, 1 horizontal, 1 perpendicular, 1 point on line
sketch "Sketch47 outline for Extrusion44" plane through (-2.54, 0, 1.734585) normal (1, 0, 0) x (0, 0, -1)
  line L0 (-10.965415, 2.54) -> (-10.965415, -1.27)
  line L1 (-3.091415, 2.54) -> (-10.965415, 2.54)
  line L2 (-10.965415, -1.27) -> (-3.091415, 2.54)
extrude "Extrusion44" cut sketch "Sketch47 outline for Extrusion44" against normal blind 25.4
sketch "Sketch49" plane through (0, -1.27, 0) normal (0, -1, 0) x (1, 0, 0)
  line L0 (-8.255, 4.826) -> (-4.445, 4.826)
  line L1 (-2.54, 1.734585) -> (-2.54, 12.7)
  line L2 (-5.498457, 4.826) -> (-2.54, 4.826)
  line L3 (-2.54, 4.826) -> (-2.54, 6.096)
  line L4 (-2.54, 6.096) -> (-5.498457, 6.096)
  line L5 (-5.498457, 6.096) -> (-5.498457, 4.826)
  point P0 (0, 0)
  dimension "d123" = 1.27
  constraints: 8 end point, 2 parallel, 2 point on line, 1 horizontal, 1 perpendicular
  measures "d123" distance of L3.end L2.end
sketch "Sketch49 outline for Extrusion46" plane through (0, -1.27, 0) normal (0, -1, 0) x (1, 0, 0)
  line L0 (-5.498457, 6.096) -> (-5.498457, 4.826)
  line L1 (-2.54, 6.096) -> (-5.498457, 6.096)
  line L2 (-2.54, 4.826) -> (-2.54, 6.096)
  line L3 (-4.445, 4.826) -> (-2.54, 4.826)
  line L4 (-5.498457, 4.826) -> (-4.445, 4.826)
extrude "Extrusion46" add sketch "Sketch49 outline for Extrusion46" along normal blind 1.27
sketch "Sketch50" plane through (-5.462315, -1.27, 6.096) normal (0, 0, 1) x (1, 0, 0)
  line L0 (0, 0) -> (2.032, 0)
  line L1 (2.032, 0) -> (2.032, -0.762)
  line L2 (2.032, -0.762) -> (0, -0.762)
  line L3 (0, -0.762) -> (0, 0)
  point P0 (5.462315, 1.27)
  dimension "d126" = 2.032
  dimension "d127" = 0.762
  constraints: 8 end point, 2 parallel, 1 horizontal, 1 perpendicular
  measures "d126" distance of L1.end L2.end
  measures "d127" distance of L0.end L1.end
sketch "Sketch50 outline for Extrusion47" plane through (-5.462315, -1.27, 6.096) normal (0, 0, 1) x (1, 0, 0)
  line L0 (0, 0) -> (0, -0.762)
  line L1 (2.032, 0) -> (0, 0)
  line L2 (2.032, -0.762) -> (2.032, 0)
  line L3 (0, -0.762) -> (2.032, -0.762)
extrude "Extrusion47" cut sketch "Sketch50 outline for Extrusion47" against normal blind 1.27
sketch "Sketch51" plane through (0, -1.27, 0) normal (0, -1, 0) x (1, 0, 0)
  circle A0 centre (-8.255, 10.23115) radius 1.016
  point P0 (0, 0)
  dimension "d130" = 2.032
  constraints: 1 centre point
  measures "d130" diameter of A0
sketch "Sketch51 outline for Extrusion48" plane through (0, -1.27, 0) normal (0, -1, 0) x (1, 0, 0)
  circle A0 centre (-8.255, 10.23115) radius 1.016
extrude "Extrusion48" cut sketch "Sketch51 outline for Extrusion48" against normal blind 25.4
sketch "Sketch52" plane through (-6.35, 2.54, -20.32) normal (0, -1, 0) x (1, 0, 0)
  circle A0 centre (0, 0) radius 4.445 projected
  circle A1 centre (0, 0) radius 4.445
  point P0 (6.35, 20.32)
  constraints: 1 centre point, 1 coincident
sketch "Sketch52 outline for Extrusion49" plane through (-6.35, 2.54, -20.32) normal (0, -1, 0) x (1, 0, 0)
  circle A0 centre (0, 0) radius 4.445
extrude "Extrusion49" cut sketch "Sketch52 outline for Extrusion49" against normal blind 1.27
sketch "Sketch53" plane through (-6.35, 3.81, -8.89) normal (0, -1, 0) x (1, 0, 0)
  circle A0 centre (0, 0) radius 4.445 projected
  circle A1 centre (0, 0) radius 1.905
  circle A2 centre (0, -11.43) radius 4.445 projected
  circle A3 centre (0, -11.43) radius 1.905
  point P0 (6.35, 8.89)
  dimension "d135" = 3.81
  dimension "d136" = 3.81
  constraints: 2 centre point, 2 coincident
  measures "d135" diameter of A1
  measures "d136" diameter of A3
sketch "Sketch53 outline for Extrusion50" plane through (-6.35, 3.81, -8.89) normal (0, -1, 0) x (1, 0, 0)
  circle A0 centre (0, 0) radius 1.905
  circle A1 centre (0, -11.43) radius 1.905
extrude "Extrusion50" cut sketch "Sketch53 outline for Extrusion50" against normal blind 25.4
sketch "Sketch54" plane through (0.254, 0, -25.4) normal (1, 0, 0) x (0, 0, -1)
  line L0 (0, 10.16) -> (-17.78, 10.16)
  line L1 (0, 10.16) -> (-31.24915, 10.16)
  line L2 (-31.24915, 10.16) -> (-31.24915, 5.08)
  line L3 (-31.24915, 5.08) -> (0, 5.08)
  line L4 (0, 5.08) -> (0, 10.16)
  point P0 (-25.4, 0)
  dimension "d139" = 5.08
  constraints: 8 end point, 2 parallel, 1 horizontal, 1 perpendicular
  measures "d139" distance of L2.end L1.end
sketch "Sketch54 outline for Extrusion51" plane through (0.254, 0, -25.4) normal (1, 0, 0) x (0, 0, -1)
  line L0 (0, 5.08) -> (0, 10.16)
  line L1 (-31.24915, 5.08) -> (0, 5.08)
  line L2 (-31.24915, 10.16) -> (-31.24915, 5.08)
  line L3 (-17.78, 10.16) -> (-31.24915, 10.16)
  line L4 (0, 10.16) -> (-17.78, 10.16)
extrude "Extrusion51" cut sketch "Sketch54 outline for Extrusion51" against normal blind 25.4
sketch "Sketch55" plane through (0, -1.27, 0) normal (0, -1, 0) x (1, 0, 0)
  line L0 (-2.54, 4.826) -> (-2.54, -2.54)
  line L1 (-2.54, 4.826) -> (-3.429, 4.826)
  line L2 (-3.429, 4.826) -> (-3.429, 2.501434)
  line L3 (-3.429, 2.501434) -> (-2.54, 2.501434)
  line L4 (-2.54, 2.501434) -> (-2.54, 4.826)
  line L5 (-10.16, 1.734585) -> (-2.54, 1.734585)
  line L6 (-2.54, 1.734585) -> (-2.54, 2.501434)
  line L7 (-2.54, 2.501434) -> (-10.16, 2.501434)
  line L8 (-10.16, 2.501434) -> (-10.16, 1.734585)
  line L9 (-7.300103, 12.7) -> (-10.16, 12.7)
  line L10 (-10.16, 2.501434) -> (-9.295399, 2.501434)
  line L11 (-9.295399, 2.501434) -> (-9.295399, 12.7)
  line L12 (-9.295399, 12.7) -> (-10.16, 12.7)
  line L13 (-10.16, 12.7) -> (-10.16, 2.501434)
  point P0 (0, 0)
  dimension "d142" = 0.8646
  dimension "d143" = 0.889
  constraints: 24 end point, 6 parallel, 3 horizontal, 3 perpendicular, 1 point on line
  measures "d142" distance of L11.end L9.end
  measures "d143" distance of L3.end L2.end
sketch "Sketch55 outline for Extrusion52" plane through (0, -1.27, 0) normal (0, -1, 0) x (1, 0, 0)
  line L0 (-10.16, 12.7) -> (-10.16, 2.501434)
  line L1 (-9.295399, 12.7) -> (-10.16, 12.7)
  line L2 (-9.295399, 2.501434) -> (-9.295399, 12.7)
  line L3 (-3.429, 2.501434) -> (-9.295399, 2.501434)
  line L4 (-3.429, 4.826) -> (-3.429, 2.501434)
  line L5 (-2.54, 4.826) -> (-3.429, 4.826)
  line L6 (-2.54, 1.734585) -> (-2.54, 4.826)
  line L7 (-10.16, 1.734585) -> (-2.54, 1.734585)
  line L8 (-10.16, 2.501434) -> (-10.16, 1.734585)
extrude "Extrusion52" add sketch "Sketch55 outline for Extrusion52" along normal blind 1.27
sketch "Sketch56" plane through (-3.430315, -2.032, 4.826) normal (0, 0, -1) x (-1, 0, 0)
  line L0 (2.032, -0.508) -> (-0.001315, -0.508)
  line L1 (0, 0) -> (0, 0.762)
  line L2 (-0.001315, -0.508) -> (0, -0.508)
  line L3 (0, -0.508) -> (0, 0)
  line L4 (0, 0) -> (-0.001315, 0)
  line L5 (-0.001315, 0) -> (-0.001315, -0.508)
  line L6 (2.032, 0) -> (0, 0)
  line L7 (2.032, 0) -> (0, 0)
  line L8 (0, 0) -> (0, -0.508)
  line L9 (0, -0.508) -> (2.032, -0.508)
  line L10 (2.032, -0.508) -> (2.032, 0)
  point P0 (-3.430315, 2.032)
  constraints: 16 end point, 4 parallel, 2 horizontal, 2 perpendicular
sketch "Sketch56 outline for Extrusion53" plane through (-3.430315, -2.032, 4.826) normal (0, 0, -1) x (-1, 0, 0)
  line L0 (2.032, -0.508) -> (2.032, 0)
  line L1 (0, -0.508) -> (2.032, -0.508)
  line L2 (0, 0) -> (0, -0.508)
  line L3 (2.032, 0) -> (0, 0)
extrude "Extrusion53" add sketch "Sketch56 outline for Extrusion53" along normal blind 2.54
sketch "Sketch57" plane through (-5.462315, -2.54, 6.096) normal (0, 0, 1) x (1, 0, 0)
  line L0 (2.922315, 0) -> (0, 0)
  line L1 (2.032, 1.27) -> (2.922315, 1.27)
  line L2 (2.922315, 1.27) -> (2.922315, 0)
  line L3 (2.922315, 0) -> (2.032, 0)
  line L4 (2.032, 0) -> (2.032, 1.27)
  line L5 (2.032, 0.508) -> (0, 0.508)
  line L6 (0.001315, 0) -> (2.032, 0)
  line L7 (2.032, 0) -> (2.032, 0.508)
  line L8 (2.032, 0.508) -> (0.001315, 0.508)
  line L9 (0.001315, 0.508) -> (0.001315, 0)
  point P0 (5.462315, 2.54)
  constraints: 16 end point, 4 parallel, 2 horizontal, 2 perpendicular, 1 point on line
sketch "Sketch57 outline for Extrusion54" plane through (-5.462315, -2.54, 6.096) normal (0, 0, 1) x (1, 0, 0)
  line L0 (2.922315, 0) -> (2.922315, 1.27)
  line L1 (0.001315, 0) -> (2.922315, 0)
  line L2 (0.001315, 0.508) -> (0.001315, 0)
  line L3 (2.032, 0.508) -> (0.001315, 0.508)
  line L4 (2.032, 1.27) -> (2.032, 0.508)
  line L5 (2.922315, 1.27) -> (2.032, 1.27)
extrude "Extrusion54" add sketch "Sketch57 outline for Extrusion54" along normal blind 3.556
sketch "Sketch59" plane through (0, -2.54, 0) normal (0, -1, 0) x (1, 0, 0)
  line L0 (-5.461, 2.501434) -> (-3.429, 2.501434)
  line L1 (-3.430315, 9.652) -> (-5.461, 9.652)
  line L2 (-4.572, 2.501434) -> (-4.064, 2.501434)
  line L3 (-4.064, 2.501434) -> (-4.064, 9.652)
  line L4 (-4.064, 9.652) -> (-4.572, 9.652)
  line L5 (-4.572, 9.652) -> (-4.572, 2.501434)
  line L6 (-2.54, 1.734585) -> (-2.54, 9.652)
  point P0 (0, 0)
  dimension "d153" = 0.508
  dimension "d154" = 1.524
  constraints: 8 end point, 2 parallel, 2 point on line, 1 horizontal, 1 perpendicular
  measures "d153" distance of L4.end L3.end
  measures "d154" distance between parallel lines of L3 L6
sketch "Sketch59 outline for Extrusion56" plane through (0, -2.54, 0) normal (0, -1, 0) x (1, 0, 0)
  line L0 (-4.572, 9.652) -> (-4.572, 2.501434)
  line L1 (-4.064, 9.652) -> (-4.572, 9.652)
  line L2 (-4.064, 2.501434) -> (-4.064, 9.652)
  line L3 (-4.572, 2.501434) -> (-4.064, 2.501434)
extrude "Extrusion56" cut sketch "Sketch59 outline for Extrusion56" against normal blind 0.508
body "Solid1"
